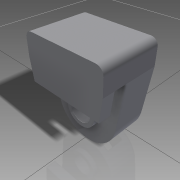
# Autodesk Inventor part: HexSaver01
Saved by Autodesk Inventor 2013 (Build 170138000, 138)
## iProperties
Created: 2014-07-22
Part Number: HexSaver01
Material: Generic
Document SubType Name: Modeling
Designer: spichelh
Density: 1 g/cm^3
Author: spichelh
Autodesk Inventor part; units mm, degrees
ref_plane "YZ Plane" through (0, 0, 0) normal (1, 0, 0) x (0, 1, 0)
ref_plane "XZ Plane" through (0, 0, 0) normal (0, 1, 0) x (-1, 0, 0)
ref_plane "XY Plane" through (0, 0, 0) normal (0, 0, 1) x (1, 0, 0)
sketch "Sketch1" plane through (0, 0, 0) normal (0, 0, 1) x (1, 0, 0)
  circle A0 centre (0, 0) radius 1
  line L0 (-8.2702, 3.81) -> (10.8086, 3.81) construction
  arc A1 (-2.9768, -0.3724) -> (2.9768, -0.3724) centre (0, 0) ccw
  line L1 (0, 0) -> (2.9768, -0.3724) construction
  line L2 (-3.5, 3.81) -> (-3.5, 5.81)
  line L3 (-3.5, 5.81) -> (3.5, 5.81)
  line L4 (3.5, 5.81) -> (3.5, 3.81)
  line L5 (0, 5.81) -> (0, -5.1474) construction
  line L6 (2.9768, -0.3724) -> (3.5, 3.81)
  line L7 (-2.9768, -0.3724) -> (-3.5, 3.81)
  dimension "d0" = 2
  dimension "d3" = 3.81
  dimension "d4" = 2
  dimension "d5" = 7
  dimension "d6" = 3
  constraints: 16 end point, 5 perpendicular, 3 point on line, 2 centre point, 2 coincident, 2 point on circle, 1 horizontal, 1 line through centre, 1 midpoint, 1 symmetric about line
  measures "d0" diameter of A0
  measures "d3" distance from line of L0 point (0, 0)
  measures "d4" distance of L2.start L2.end
  measures "d5" distance of L2.end L3.end
  measures "d6" radius of A1
extrude "Extrusion1" add sketch "Sketch1" along normal blind 5
sketch "Sketch2" plane through (3.5, 3.81, 0) normal (1, 0, 0) x (0, 0, -1)
  line L0 (-5, 0) -> (-5, 2) projected
  line L1 (0, 0) -> (-5, 0) projected
  line L2 (-4, 0) -> (-3, 0)
  line L3 (-3, 0) -> (-3, -8)
  line L4 (-3, -8) -> (-4, -8)
  line L5 (-4, -8) -> (-4, 0)
  point P0 (0, -3.81)
  dimension "d7" = 1
  dimension "d9" = 1
  dimension "d10" = 8
  constraints: 8 end point, 2 parallel, 1 horizontal, 1 perpendicular, 1 point on line
  measures "d7" distance of L3.end L4.end
  measures "d9" distance between parallel lines of L0 L5
  measures "d10" distance between parallel lines of L1 L4
extrude "Extrusion2" cut sketch "Sketch2" against normal blind 10
sketch "Sketch3" plane through (0, 0, 3) normal (0, 0, 1) x (1, 0, 0)
  arc A0 (-2.9768, -0.3724) -> (2.9768, -0.3724) centre (0, 0) ccw projected
  line L0 (3.5, 3.81) -> (-3.5, 3.81) projected
  circle A1 centre (0, 0) radius 1 projected
  line L1 (0, 2.3094) -> (2, 1.1547)
  line L2 (2, 1.1547) -> (2, -1.1547)
  line L3 (2, -1.1547) -> (0, -2.3094)
  line L4 (0, -2.3094) -> (-2, -1.1547)
  line L5 (-2, -1.1547) -> (-2, 1.1547)
  line L6 (-2, 1.1547) -> (0, 2.3094)
  line L7 (0, 3.81) -> (0, 1.7188) construction
  point P0 (0, 0)
  dimension "d13" = 2
  constraints: 14 end point, 1 coincident, 1 midpoint, 1 parallel, 1 point on line, 13 other
  measures "d13" distance from line of L1 A0.centre
extrude "Extrusion3" cut sketch "Sketch3" against normal blind 2.5
sketch "Sketch5" plane through (0, 0, 3) normal (0, 0, 1) x (1, 0, 0)
  line L0 (-2, 1.1547) -> (0, 2.3094) projected
  line L1 (0, 2.3094) -> (2, 1.1547) projected
  line L2 (2, 1.1547) -> (2, -1.1547) projected
  line L3 (2, -1.1547) -> (0, -2.3094) projected
  line L4 (0, -2.3094) -> (-2, -1.1547) projected
  line L5 (-2, -1.1547) -> (-2, 1.1547) projected
  circle A0 centre (0, 0) radius 1 projected
extrude "Extrusion5" add sketch "Sketch5" against normal blind 0.5
ref_plane "Work Plane1" through (-3.5, -2.69, 0) normal (0, 1, 0) x (1, 0, 0)
sketch "Sketch6" plane through (-3.5, -2.69, 0) normal (0, 1, 0) x (1, 0, 0)
  line L0 (1.5, -2.5) -> (3.5, -2.5) projected
  line L1 (3.5, -2.5) -> (3.5, -0.5) projected
  line L2 (1.5, -2.5) -> (1.5, -0.5) projected
  line L3 (3.5, -2.5) -> (5.5, -2.5) projected
  line L4 (5.5, -2.5) -> (5.5, -0.5) projected
  line L5 (3.5, -2.5) -> (3.5, -0.5) projected
  line L6 (5.4, -0.6) -> (1.6, -0.6)
  line L7 (1.6, -0.6) -> (1.6, -2.4)
  line L8 (1.6, -2.4) -> (5.4, -2.4)
  line L9 (5.4, -2.4) -> (5.4, -0.6)
  line L10 (5.5, -0.5) -> (3.5, -0.5) projected
  line L11 (3.5, -0.5) -> (1.5, -0.5) projected
  point P0 (3.5, 0)
  dimension "d28" = 0.1
  dimension "d29" = 0.1
  dimension "d30" = 0.1
  constraints: 8 end point, 2 parallel, 1 horizontal, 1 perpendicular
  measures "d28" distance between parallel lines of L3 L8
  measures "d29" distance between parallel lines of L9 L4
  measures "d30" distance between parallel lines of L2 L7
extrude "Extrusion6" cut sketch "Sketch6" along normal blind 2 and the other way blind 2 contours L8 L7 L6 L1 | L1 L6 L9 L8
sketch "Sketch7" plane through (0, 0, 5) normal (0, 0, 1) x (1, 0, 0)
  circle A0 centre (0, 0) radius 1 projected
  arc A1 (-2.9768, -0.3724) -> (2.9768, -0.3724) centre (0, 0) ccw projected
  line L0 (2.9768, -0.3724) -> (3.5, 3.81) projected
  line L1 (3.5, 3.81) -> (3.5, 5.21) projected
  line L2 (2.9, 5.81) -> (-2.9, 5.81) projected
  line L3 (-3.5, 5.21) -> (-3.5, 3.81) projected
  line L4 (-3.5, 3.81) -> (-2.9768, -0.3724) projected
  line L5 (-3.5, 3.81) -> (3.5, 3.81)
  arc A2 (-2.9, 5.81) -> (-3.5, 5.21) centre (-2.9, 5.21) ccw projected
  arc A3 (3.5, 5.21) -> (2.9, 5.81) centre (2.9, 5.21) ccw projected
  line L6 (2.9768, -0.3724) -> (3.5, 3.81) projected
  line L7 (-3.5, 5.81) -> (-3.5, 3.81) projected
  line L8 (-3.5, 3.81) -> (-2.9768, -0.3724) projected
  line L9 (-3.2498, 1.81) -> (3.2498, 1.81)
  dimension "d35" = 2
  constraints: 4 end point, 2 perpendicular, 2 point on line
  measures "d35" distance between parallel lines of L5 L9
fillet "Fillet1" radius 0.6 2 edges at (3.5, 5.81, 2.5) (-3.5, 5.81, 2.5)
extrude "Extrusion7" cut sketch "Sketch7" against normal blind 2 contours L4 L9 L0 A1
sketch "Sketch8" plane through (0, 0, 3) normal (0, 0, 1) x (1, 0, 0)
  circle A0 centre (0, 0) radius 1 projected
  arc A1 (-2.9768, -0.3724) -> (2.9768, -0.3724) centre (0, 0) ccw projected
  circle A2 centre (0, 0) radius 1.4
  circle A3 centre (0, 0) radius 1
  dimension "d36" = 2.8
  dimension "d37" = 2
  constraints: 2 centre point, 2 coincident
  measures "d36" diameter of A2
  measures "d37" diameter of A3
extrude "Extrusion8" add sketch "Sketch8" along normal blind 0.5
body "Solid1"
